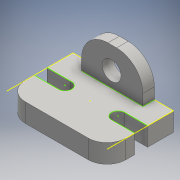
# Autodesk Inventor part: 240531_3Dsketch01
Saved by Autodesk Inventor 2016 (Build 200138000, 138)
## iProperties
Created: 2024-05-31
Part Number: 240531_3Dsketch01
Material: 일반
Document SubType Name: Modeling
Designer: pc
Density: 1 g/cm^3
Appearance: 기본값
Author: pc
Autodesk Inventor part; units mm, degrees
ref_plane "YZ Plane" through (0, 0, 0) normal (1, 0, 0) x (0, 1, 0)
ref_plane "XZ Plane" through (0, 0, 0) normal (0, 1, 0) x (-1, 0, 0)
ref_plane "XY Plane" through (0, 0, 0) normal (0, 0, 1) x (1, 0, 0)
sketch "스케치1" plane through (0, 0, 0) normal (0, 0, 1) x (1, 0, 0)
  line L0 (13.3752, -8.8292) -> (-13.3752, -8.8292)
  line L1 (-13.3752, -8.8292) -> (-13.3752, 8.8292)
  line L2 (-13.3752, 8.8292) -> (13.3752, 8.8292)
  line L3 (13.3752, 8.8292) -> (13.3752, -8.8292)
  line L4 (13.3752, -8.8292) -> (-13.3752, 8.8292) construction
  line L5 (-13.3752, -8.8292) -> (13.3752, 8.8292) construction
  point P0 (0, 0)
  constraints: 12 end point, 2 midpoint, 2 parallel, 1 horizontal, 1 perpendicular
extrude "돌출1" add sketch "스케치1" along normal blind 5
sketch "스케치2" plane through (0, 0, 5) normal (0, 0, 1) x (1, 0, 0)
  line L0 (13.3752, 8.8292) -> (-13.3752, 8.8292) projected
  line L1 (-8.0009, 8.8292) -> (8.3241, 8.8292)
  line L2 (8.3241, 8.8292) -> (8.3241, 5.7582)
  line L3 (8.3241, 5.7582) -> (-8.0009, 5.7582)
  line L4 (-8.0009, 5.7582) -> (-8.0009, 8.8292)
  line L5 (-13.3752, 8.8292) -> (-13.3752, -8.8292) projected
  line L6 (-13.3752, 1.9598) -> (-7.1927, 1.9598)
  line L7 (-13.3752, -1.5153) -> (-7.1927, -1.5153)
  arc A0 (-7.1927, -1.5153) -> (-7.1927, 1.9598) centre (-6.9174, 0.2222) ccw
  line L8 (13.3752, -8.8292) -> (13.3752, 8.8292) projected
  line L9 (13.3752, 1.9598) -> (7.2331, 1.9598)
  line L10 (13.3752, -1.5153) -> (7.2331, -1.5153)
  arc A1 (7.2331, 1.9598) -> (7.2331, -1.5153) centre (7.2331, 0.2222) ccw
  point P0 (0, 0)
  constraints: 16 end point, 5 horizontal, 5 point on line, 4 point on circle, 2 centre point, 2 parallel, 2 tangent, 1 perpendicular
extrude "돌출2" add sketch "스케치2" along normal blind 10 contours L2 L3 L4 L0
extrude "돌출3" cut sketch "스케치2" against normal blind 10 contours L6 A0 L7 L5 | L8 L10 A1 L9
sketch "스케치3" plane through (-8.0009, 5.7582, 5) normal (0, -1, 0) x (1, 0, 0)
  circle A0 centre (8.0009, 4.1121) radius 2.5125
  line L0 (0, 10) -> (16.325, 10) projected
  line L1 (0, 0) -> (0, 10) projected
  arc A1 (8.1625, 10) -> (0, 4.1121) centre (8.0451, 1.5609) ccw
  line L2 (16.325, 0) -> (16.325, 10) projected
  arc A2 (16.325, 4.1121) -> (8.1625, 10) centre (7.959, 1.1161) ccw
  point P0 (8.0009, -5)
  constraints: 4 point on circle, 3 centre point, 2 point on line, 1 midpoint
extrude "돌출4" cut sketch "스케치3" against normal blind 10 contours A0
fillet "모깎기1" radius 5 2 edges at (13.3752, -8.8292, 2.5) (-13.3752, -8.8292, 2.5)
sketch "스케치4" plane through (-8.0009, 5.7582, 5) normal (0, -1, 0) x (1, 0, 0)
  point P0 (8.0009, -5)
fillet "모깎기2" radius 7 2 edges at (8.3241, 7.2937, 15) (-8.0009, 7.2937, 15)
